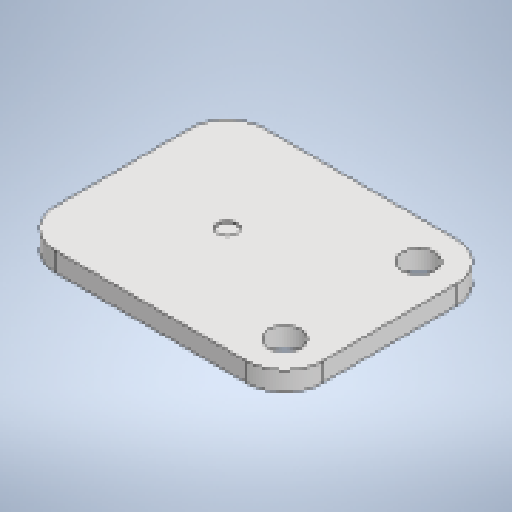
# Autodesk Inventor part: PNS-683 leg floor plate
Saved by Autodesk Inventor 2025 (Build 290162010, 162A)
## iProperties
Created: 2025-02-20
Part Number: PNS-683 leg floor plate
Material: Stainless Steel
Document SubType Name: Sheet Metal
Designer: admin
Mass: 1070.67 g
Surface Area: 320.872 cm^2
Volume: 133.833 cm^3
Density: 8 g/cm^3
Sheet Metal Rule: AISI304 3mm Die 32
Sheet Metal Width: 110,000 mm
Sheet Metal Length: 140,000 mm
Sheet Metal Area: 15400,000 mm^2
Appearance: Default
Flat Pattern Width: 11 cm
Flat Pattern Length: 14 cm
Flat Pattern Area: 154 cm^2
Author: user
Autodesk Inventor part; units mm, degrees
ref_plane "YZ Plane" through (0, 0, 0) normal (1, 0, 0) x (0, 1, 0)
ref_plane "XZ Plane" through (0, 0, 0) normal (0, 1, 0) x (-1, 0, 0)
ref_plane "XY Plane" through (0, 0, 0) normal (0, 0, 1) x (1, 0, 0)
sketch "Sketch1" plane through (0, 0, 0) normal (0, 0, 1) x (1, 0, 0)
  line L0 (-70, -55) -> (70, -55)
  line L1 (70, -55) -> (70, 55)
  line L2 (70, 55) -> (-70, 55)
  line L3 (-70, 55) -> (-70, -55)
  line L4 (-70, -55) -> (70, 55) construction
  line L5 (70, -55) -> (-70, 55) construction
  circle A0 centre (50, -35) radius 8.5
  circle A1 centre (50, 35) radius 8.5
  line L6 (0, 0) -> (70, 0) construction
  circle A2 centre (50, 0) radius 8.5
  dimension "d0" = 140
  dimension "d1" = 110
  dimension "d23" = 17
  dimension "d25" = 20
  dimension "d26" = 20
  measures "d0" distance of L2.end L1.end
  measures "d1" distance of L1.end L0.end
  measures "d23" diameter of A0
  measures "d25" distance from line of L1 A0.centre
  measures "d26" distance from line of A0.centre L0
extrude "Plate1" add sketch "Sketch1" along normal blind 6 contours L3 L2 L1 L0 | A0 | A1
sketch "Sketch5" plane through (0, 0, 6) normal (0, 0, 1) x (1, 0, 0)
  line L0 (70, -55) -> (-70, -55) projected
  line L1 (-70, -55) -> (-70, 55) projected
  line L2 (-70, 55) -> (70, 55) projected
  circle A0 centre (-15, 0) radius 55
  circle A1 centre (-15, 0) radius 5
  point P0 (0, 0)
  point P1 (50, -55)
  point P2 (-50, -55)
  point P3 (-70, -35)
  point P4 (-70, 35)
  point P5 (-50, 55)
  point P6 (50, 55)
  dimension "d27" = 10
  constraints: 3 tangent, 2 centre point, 1 coincident
  measures "d27" diameter of A1
extrude "Extrusion2" cut sketch "Sketch5" against normal blind 1 contours A1
chamfer "Corner Chamfer2" distance 30 angle 45 2 edges at (70, -55, 3) (70, 55, 3)
fillet "Corner Round2" radius 6 6 edges at (40, -55, 3) (70, -25, 3) (70, 25, 3) (40, 55, 3) (-70, 55, 3) (-70, -55, 3)
equation "\"d26\" = d25"
equation "\"d2\" = Thickness"
equation "\"BendReliefWidth\" = Thickness"
equation "\"BendReliefDepth\" = 0.5 * Thickness"
equation "\"CornerReliefSize\" = 4 * Thickness"
equation "\"MinimumRemnant\" = 2 * Thickness"
equation "\"TransitionRadius\" = BendRadius"
equation "\"JacobiRadiusSize\" = BendRadius"
equation "\"GapSize\" = Thickness"
equation "\"Thickness\" = 6"
equation "\"BendRadius\" = 5"
body "Solid1"
